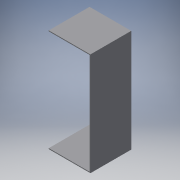
# Autodesk Inventor part: Part96
Saved by Autodesk Inventor 2016 (Build 200138000, 138)
## iProperties
Created: 2016-09-04
Part Number: Part96
Material: Generic
Document SubType Name: Modeling
Designer: gus
Density: 1 g/cm^3
Appearance: Default
Author: gus
Autodesk Inventor part; units mm, degrees
ref_plane "YZ Plane" through (0, 0, 0) normal (1, 0, 0) x (0, 1, 0)
ref_plane "XZ Plane" through (0, 0, 0) normal (0, 1, 0) x (-1, 0, 0)
ref_plane "XY Plane" through (0, 0, 0) normal (0, 0, 1) x (1, 0, 0)
sketch "Sketch1" plane through (0, 0, 0) normal (0, 0, 1) x (1, 0, 0)
  line L0 (0, 0) -> (-3.175, 0)
  line L1 (-3.175, 0) -> (-3.175, -384.175)
  line L2 (-3.175, -384.175) -> (0, -384.175)
  line L3 (0, -384.175) -> (0, 0)
  dimension "d0" = 3.175
  dimension "d1" = 384.175
  constraints: 8 end point, 2 parallel, 1 horizontal, 1 perpendicular
  measures "d0" distance of L2.end L1.end
  measures "d1" distance of L1.end L0.end
extrude "Extrusion1" add sketch "Sketch1" along normal blind 152.4
sketch "Sketch2" plane through (-3.175, -384.175, 0) normal (-1, 0, 0) x (0, 0, 1)
  line L0 (0, 384.175) -> (0, 0) projected
  line L1 (152.4, 384.175) -> (0, 384.175)
  line L2 (0, 384.175) -> (0, 381)
  line L3 (0, 381) -> (152.4, 381)
  line L4 (152.4, 381) -> (152.4, 384.175)
  line L5 (0, 384.175) -> (152.4, 384.175) projected
  line L6 (152.4, 384.175) -> (152.4, 0) projected
  line L7 (152.4, 0) -> (0, 0)
  line L8 (0, 0) -> (0, 3.175)
  line L9 (0, 3.175) -> (152.4, 3.175)
  line L10 (152.4, 3.175) -> (152.4, 0)
  dimension "d4" = 152.4
  dimension "d5" = 3.175
  dimension "d6" = 3.175
  constraints: 16 end point, 4 parallel, 2 horizontal, 2 perpendicular, 2 point on line, 1 collinear
  measures "d4" distance of L2.end L3.end
  measures "d5" distance of L3.end L1.start
  measures "d6" distance between parallel lines of L9 L7
extrude "Extrusion2" add sketch "Sketch2" along normal blind 152.4 contours L1 L4 L3 L0 | L9 L6 L7 L0
sketch "Sketch3" plane through (0, -384.175, 0) normal (0, -1, 0) x (1, 0, 0)
  line L0 (-3.175, 152.4) -> (49.7899, 295.3003)
  line L1 (49.7899, 295.3003) -> (52.767, 294.1968)
  line L2 (52.767, 294.1968) -> (-0.1979, 151.2966)
  line L3 (-0.1979, 151.2966) -> (-3.175, 152.4)
  point P0 (0, 0)
  dimension "d9" = 3.175
  dimension "d10" = 152.4
  constraints: 8 end point, 2 parallel, 1 perpendicular
  measures "d9" distance between parallel lines of L2 L0
  measures "d10" distance of L1.end L2.end
extrude "Extrusion3" add sketch "Sketch3" against normal blind 384.175
body "Solid1"
